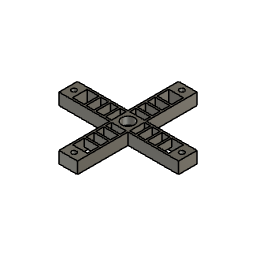
gripper v1 (Autodesk Fusion 360 design; units mm, degrees)
Autodesk Fusion 360 part; units mm, degrees
sketch "Esboço1" plane through (0, 0, 0) normal (0, 0, 1) x (1, 0, 0)
  line L0 (9.5, 9.5) -> (-9.5, 9.5)
  line L1 (-9.5, 9.5) -> (-9.5, -9.5)
  line L2 (-9.5, -9.5) -> (9.5, -9.5)
  line L3 (9.5, -9.5) -> (9.5, 9.5)
  line L4 (9.5, 9.5) -> (-9.5, -9.5) construction
  line L5 (-9.5, 9.5) -> (9.5, -9.5) construction
  circle A0 centre (0, 0) radius 6.5
  line L6 (-9.5, 9.5) -> (-7.5, 9.5)
  line L7 (-7.5, 9.5) -> (-7.5, 7.5)
  line L8 (-7.5, 7.5) -> (-9.5, 7.5)
  line L9 (-9.5, 7.5) -> (-9.5, 9.5)
  line L10 (9.5, 9.5) -> (7.5, 9.5)
  line L11 (7.5, 9.5) -> (7.5, 7.5)
  line L12 (7.5, 7.5) -> (9.5, 7.5)
  line L13 (9.5, 7.5) -> (9.5, 9.5)
  line L14 (-9.5, -9.5) -> (-7.5, -9.5)
  line L15 (-7.5, -9.5) -> (-7.5, -7.5)
  line L16 (-7.5, -7.5) -> (-9.5, -7.5)
  line L17 (-9.5, -7.5) -> (-9.5, -9.5)
  line L18 (9.5, -9.5) -> (7.5, -9.5)
  line L19 (7.5, -9.5) -> (7.5, -7.5)
  line L20 (7.5, -7.5) -> (9.5, -7.5)
  line L21 (9.5, -7.5) -> (9.5, -9.5)
  line L22 (-9.5, 9.5) -> (-7.5, 9.5)
  line L23 (-7.5, 9.5) -> (-7.5, 49.5)
  line L24 (-7.5, 49.5) -> (-9.5, 49.5)
  line L25 (-9.5, 49.5) -> (-9.5, 9.5)
  line L26 (9.5, 9.5) -> (7.5, 9.5)
  line L27 (7.5, 9.5) -> (7.5, 49.5)
  line L28 (7.5, 49.5) -> (9.5, 49.5)
  line L29 (9.5, 49.5) -> (9.5, 9.5)
  line L30 (-9.5, 49.5) -> (9.5, 49.5)
  line L31 (9.5, 49.5) -> (9.5, 61.5)
  line L32 (9.5, 61.5) -> (-9.5, 61.5)
  line L33 (-9.5, 61.5) -> (-9.5, 49.5)
  line L34 (-9.5, 61.5) -> (9.5, 49.5) construction
  circle A1 centre (0, 55.5) radius 2.5
  line L35 (-7.5, 9.5) -> (7.5, 9.5)
  line L36 (7.5, 9.5) -> (7.5, 15.5)
  line L37 (7.5, 15.5) -> (-7.5, 15.5)
  line L38 (-7.5, 15.5) -> (-7.5, 9.5)
  line L39 (-7.5, 15.5) -> (7.5, 15.5)
  line L40 (7.5, 15.5) -> (7.5, 17.5)
  line L41 (7.5, 17.5) -> (-7.5, 17.5)
  line L42 (-7.5, 17.5) -> (-7.5, 15.5)
  line L43 (-7.5, 17.5) -> (7.5, 17.5)
  line L44 (7.5, 17.5) -> (7.5, 25.5)
  line L45 (7.5, 25.5) -> (-7.5, 25.5)
  line L46 (-7.5, 25.5) -> (-7.5, 17.5)
  line L47 (-7.5, 25.5) -> (7.5, 25.5)
  line L48 (7.5, 25.5) -> (7.5, 27.5)
  line L49 (7.5, 27.5) -> (-7.5, 27.5)
  line L50 (-7.5, 27.5) -> (-7.5, 25.5)
  line L51 (-7.5, 27.5) -> (7.5, 27.5)
  line L52 (7.5, 27.5) -> (7.5, 35.5)
  line L53 (7.5, 35.5) -> (-7.5, 35.5)
  line L54 (-7.5, 35.5) -> (-7.5, 27.5)
  line L55 (-7.5, 35.5) -> (7.5, 35.5)
  line L56 (7.5, 35.5) -> (7.5, 37.5)
  line L57 (7.5, 37.5) -> (-7.5, 37.5)
  line L58 (-7.5, 37.5) -> (-7.5, 35.5)
  line L59 (9.5, 9.5) -> (49.5, 9.5)
  line L60 (49.5, 9.5) -> (49.5, 7.5)
  line L61 (49.5, 7.5) -> (9.5, 7.5)
  line L62 (9.5, 7.5) -> (9.5, 9.5)
  line L63 (9.5, -9.5) -> (49.5, -9.5)
  line L64 (49.5, -9.5) -> (49.5, -7.5)
  line L65 (49.5, -7.5) -> (9.5, -7.5)
  line L66 (9.5, -7.5) -> (9.5, -9.5)
  line L67 (49.5, 9.5) -> (61.5, 9.5)
  line L68 (61.5, 9.5) -> (61.5, -9.5)
  line L69 (61.5, -9.5) -> (49.5, -9.5)
  line L70 (49.5, -9.5) -> (49.5, 9.5)
  line L71 (49.5, 9.5) -> (61.5, -9.5) construction
  circle A2 centre (55.5, 0) radius 2.5
  line L72 (9.5, 7.5) -> (15.5, 7.5)
  line L73 (15.5, 7.5) -> (15.5, -7.5)
  line L74 (15.5, -7.5) -> (9.5, -7.5)
  line L75 (9.5, -7.5) -> (9.5, 7.5)
  line L76 (15.5, 7.5) -> (17.5, 7.5)
  line L77 (17.5, 7.5) -> (17.5, -7.5)
  line L78 (17.5, -7.5) -> (15.5, -7.5)
  line L79 (15.5, -7.5) -> (15.5, 7.5)
  line L80 (17.5, 7.5) -> (25.5, 7.5)
  line L81 (25.5, 7.5) -> (25.5, -7.5)
  line L82 (25.5, -7.5) -> (17.5, -7.5)
  line L83 (17.5, -7.5) -> (17.5, 7.5)
  line L84 (25.5, 7.5) -> (27.5, 7.5)
  line L85 (27.5, 7.5) -> (27.5, -7.5)
  line L86 (27.5, -7.5) -> (25.5, -7.5)
  line L87 (25.5, -7.5) -> (25.5, 7.5)
  line L88 (27.5, 7.5) -> (35.5, 7.5)
  line L89 (35.5, 7.5) -> (35.5, -7.5)
  line L90 (35.5, -7.5) -> (27.5, -7.5)
  line L91 (27.5, -7.5) -> (27.5, 7.5)
  line L92 (35.5, 7.5) -> (37.5, 7.5)
  line L93 (37.5, 7.5) -> (37.5, -7.5)
  line L94 (37.5, -7.5) -> (35.5, -7.5)
  line L95 (35.5, -7.5) -> (35.5, 7.5)
  line L96 (-9.5, -9.5) -> (-7.5, -9.5)
  line L97 (-7.5, -9.5) -> (-7.5, -49.5)
  line L98 (-7.5, -49.5) -> (-9.5, -49.5)
  line L99 (-9.5, -49.5) -> (-9.5, -9.5)
  line L100 (9.5, -9.5) -> (7.5, -9.5)
  line L101 (7.5, -9.5) -> (7.5, -49.5)
  line L102 (7.5, -49.5) -> (9.5, -49.5)
  line L103 (9.5, -49.5) -> (9.5, -9.5)
  line L104 (-9.5, -49.5) -> (9.5, -49.5)
  line L105 (9.5, -49.5) -> (9.5, -61.5)
  line L106 (9.5, -61.5) -> (-9.5, -61.5)
  line L107 (-9.5, -61.5) -> (-9.5, -49.5)
  line L108 (-9.5, -49.5) -> (9.5, -61.5) construction
  circle A3 centre (0, -55.5) radius 2.5
  line L109 (-9.5, -9.5) -> (9.5, -9.5)
  line L110 (9.5, -9.5) -> (9.5, -15.5)
  line L111 (9.5, -15.5) -> (-9.5, -15.5)
  line L112 (-9.5, -15.5) -> (-9.5, -9.5)
  line L113 (-9.5, -15.5) -> (9.5, -15.5)
  line L114 (9.5, -15.5) -> (9.5, -17.5)
  line L115 (9.5, -17.5) -> (-9.5, -17.5)
  line L116 (-9.5, -17.5) -> (-9.5, -15.5)
  line L117 (-9.5, -17.5) -> (9.5, -17.5)
  line L118 (9.5, -17.5) -> (9.5, -25.5)
  line L119 (9.5, -25.5) -> (-9.5, -25.5)
  line L120 (-9.5, -25.5) -> (-9.5, -17.5)
  line L121 (-9.5, -25.5) -> (9.5, -25.5)
  line L122 (9.5, -25.5) -> (9.5, -27.5)
  line L123 (9.5, -27.5) -> (-9.5, -27.5)
  line L124 (-9.5, -27.5) -> (-9.5, -25.5)
  line L125 (-9.5, -27.5) -> (9.5, -27.5)
  line L126 (9.5, -27.5) -> (9.5, -35.5)
  line L127 (9.5, -35.5) -> (-9.5, -35.5)
  line L128 (-9.5, -35.5) -> (-9.5, -27.5)
  line L129 (-9.5, -35.5) -> (9.5, -35.5)
  line L130 (9.5, -35.5) -> (9.5, -37.5)
  line L131 (9.5, -37.5) -> (-9.5, -37.5)
  line L132 (-9.5, -37.5) -> (-9.5, -35.5)
  line L133 (-9.5, 9.5) -> (-49.5, 9.5)
  line L134 (-49.5, 9.5) -> (-49.5, 7.5)
  line L135 (-49.5, 7.5) -> (-9.5, 7.5)
  line L136 (-9.5, 7.5) -> (-9.5, 9.5)
  line L137 (-9.5, -9.5) -> (-49.5, -9.5)
  line L138 (-49.5, -9.5) -> (-49.5, -7.5)
  line L139 (-49.5, -7.5) -> (-9.5, -7.5)
  line L140 (-9.5, -7.5) -> (-9.5, -9.5)
  line L141 (-49.5, -9.5) -> (-61.5, -9.5)
  line L142 (-61.5, -9.5) -> (-61.5, 9.5)
  line L143 (-61.5, 9.5) -> (-49.5, 9.5)
  line L144 (-49.5, 9.5) -> (-49.5, -9.5)
  line L145 (-61.5, 9.5) -> (-49.5, -9.5) construction
  circle A4 centre (-55.5, 0) radius 2.5
  line L146 (-9.5, 9.5) -> (-15.5, 9.5)
  line L147 (-15.5, 9.5) -> (-15.5, -9.5)
  line L148 (-15.5, -9.5) -> (-9.5, -9.5)
  line L149 (-9.5, -9.5) -> (-9.5, 9.5)
  line L150 (-15.5, 9.5) -> (-17.5, 9.5)
  line L151 (-17.5, 9.5) -> (-17.5, -9.5)
  line L152 (-17.5, -9.5) -> (-15.5, -9.5)
  line L153 (-15.5, -9.5) -> (-15.5, 9.5)
  line L154 (-17.5, 9.5) -> (-25.5, 9.5)
  line L155 (-25.5, 9.5) -> (-25.5, -9.5)
  line L156 (-25.5, -9.5) -> (-17.5, -9.5)
  line L157 (-17.5, -9.5) -> (-17.5, 9.5)
  line L158 (-25.5, 9.5) -> (-27.5, 9.5)
  line L159 (-27.5, 9.5) -> (-27.5, -9.5)
  line L160 (-27.5, -9.5) -> (-25.5, -9.5)
  line L161 (-25.5, -9.5) -> (-25.5, 9.5)
  line L162 (-27.5, 9.5) -> (-35.5, 9.5)
  line L163 (-35.5, 9.5) -> (-35.5, -9.5)
  line L164 (-35.5, -9.5) -> (-27.5, -9.5)
  line L165 (-27.5, -9.5) -> (-27.5, 9.5)
  line L166 (-35.5, 9.5) -> (-37.5, 9.5)
  line L167 (-37.5, 9.5) -> (-37.5, -9.5)
  line L168 (-37.5, -9.5) -> (-35.5, -9.5)
  line L169 (-35.5, -9.5) -> (-35.5, 9.5)
  dimension "d1" = 19
  dimension "d2" = 19
  dimension "d3" = 13
  dimension "d4" = 2
  dimension "d5" = 2
  dimension "d6" = 2
  dimension "d7" = 2
  dimension "d8" = 2
  dimension "d9" = 2
  dimension "d10" = 2
  dimension "d11" = 2
  dimension "d13" = 2
  dimension "d14" = 40
  dimension "d15" = 2
  dimension "d16" = 40
  dimension "d17" = 19
  dimension "d18" = 12
  dimension "d19" = 5
  dimension "d20" = 15
  dimension "d21" = 6
  dimension "d22" = 2
  dimension "d23" = 8
  dimension "d24" = 2
  dimension "d25" = 8
  dimension "d26" = 2
  dimension "d27" = 40
  dimension "d28" = 2
  dimension "d29" = 40
  dimension "d30" = 2
  dimension "d31" = 12
  dimension "d32" = 19
  dimension "d33" = 5
  dimension "d34" = 6
  dimension "d35" = 2
  dimension "d36" = 8
  dimension "d37" = 15
  dimension "d38" = 2
  dimension "d39" = 8
  dimension "d40" = 2
  dimension "d41" = 40
  dimension "d42" = 2
  dimension "d43" = 40
  dimension "d44" = 12
  dimension "d45" = 5
  dimension "d46" = 6
  dimension "d47" = 2
  dimension "d48" = 8
  dimension "d49" = 2
  dimension "d50" = 8
  dimension "d51" = 2
  dimension "d52" = 40
  dimension "d53" = 2
  dimension "d54" = 40
  dimension "d55" = 2
  dimension "d56" = 12
  dimension "d57" = 19
  dimension "d58" = 5
  dimension "d59" = 6
  dimension "d60" = 2
  dimension "d61" = 8
  dimension "d62" = 2
  dimension "d63" = 8
  dimension "d64" = 2
  constraint horizontal L0
  constraint perpendicular L0 L1
  constraint parallel L0 L2
  constraint parallel L1 L3
  constraint coincident L4 A0.centre
  constraint coincident L5 A0.centre
  constraint coincident A0.centre origin
  constraint horizontal L6
  constraint vertical L7
  constraint horizontal L8
  constraint vertical L9
  constraint horizontal L10
  constraint vertical L11
  constraint horizontal L12
  constraint vertical L13
  constraint horizontal L14
  constraint vertical L15
  constraint horizontal L16
  constraint vertical L17
  constraint horizontal L18
  constraint vertical L19
  constraint horizontal L20
  constraint vertical L21
  constraint horizontal L22
  constraint vertical L23
  constraint horizontal L24
  constraint vertical L25
  constraint horizontal L26
  constraint vertical L27
  constraint horizontal L28
  constraint vertical L29
  constraint horizontal L30
  constraint vertical L31
  constraint horizontal L32
  constraint vertical L33
  constraint midpoint L34 A1.centre
  constraint horizontal L35
  constraint vertical L36
  constraint horizontal L37
  constraint vertical L38
  constraint horizontal L39
  constraint vertical L40
  constraint horizontal L41
  constraint vertical L42
  constraint horizontal L43
  constraint vertical L44
  constraint horizontal L45
  constraint vertical L46
  constraint horizontal L47
  constraint vertical L48
  constraint horizontal L49
  constraint vertical L50
  constraint horizontal L51
  constraint vertical L52
  constraint horizontal L53
  constraint vertical L54
  constraint horizontal L55
  constraint vertical L56
  constraint horizontal L57
  constraint vertical L58
  constraint coincident L27 L56.end
  constraint horizontal L59
  constraint vertical L60
  constraint horizontal L61
  constraint vertical L62
  constraint horizontal L63
  constraint vertical L64
  constraint horizontal L65
  constraint vertical L66
  constraint horizontal L67
  constraint vertical L68
  constraint horizontal L69
  constraint vertical L70
  constraint midpoint L71 A2.centre
  constraint horizontal L72
  constraint vertical L73
  constraint horizontal L74
  constraint vertical L75
  constraint horizontal L76
  constraint vertical L77
  constraint horizontal L78
  constraint vertical L79
  constraint horizontal L80
  constraint vertical L81
  constraint horizontal L82
  constraint vertical L83
  constraint horizontal L84
  constraint vertical L85
  constraint horizontal L86
  constraint vertical L87
  constraint horizontal L88
  constraint vertical L89
  constraint horizontal L90
  constraint vertical L91
  constraint horizontal L92
  constraint vertical L93
  constraint horizontal L94
  constraint vertical L95
  constraint horizontal L96
  constraint vertical L97
  constraint horizontal L98
  constraint vertical L99
  constraint horizontal L100
  constraint vertical L101
  constraint horizontal L102
  constraint vertical L103
  constraint horizontal L104
  constraint vertical L105
  constraint horizontal L106
  constraint vertical L107
  constraint midpoint L108 A3.centre
  constraint horizontal L109
  constraint vertical L110
  constraint horizontal L111
  constraint vertical L112
  constraint horizontal L113
  constraint vertical L114
  constraint horizontal L115
  constraint vertical L116
  constraint horizontal L117
  constraint vertical L118
  constraint horizontal L119
  constraint vertical L120
  constraint horizontal L121
  constraint vertical L122
  constraint horizontal L123
  constraint vertical L124
  constraint horizontal L125
  constraint vertical L126
  constraint horizontal L127
  constraint vertical L128
  constraint horizontal L129
  constraint vertical L130
  constraint horizontal L131
  constraint vertical L132
  constraint horizontal L133
  constraint vertical L134
  constraint horizontal L135
  constraint vertical L136
  constraint horizontal L137
  constraint vertical L138
  constraint horizontal L139
  constraint vertical L140
  constraint horizontal L141
  constraint vertical L142
  constraint horizontal L143
  constraint vertical L144
  constraint midpoint L145 A4.centre
  constraint horizontal L146
  constraint vertical L147
  constraint horizontal L148
  constraint vertical L149
  constraint horizontal L150
  constraint vertical L151
  constraint horizontal L152
  constraint vertical L153
  constraint horizontal L154
  constraint vertical L155
  constraint horizontal L156
  constraint vertical L157
  constraint horizontal L158
  constraint vertical L159
  constraint horizontal L160
  constraint vertical L161
  constraint horizontal L162
  constraint vertical L163
  constraint horizontal L164
  constraint vertical L165
  constraint horizontal L166
  constraint vertical L167
  constraint horizontal L168
  constraint vertical L169
  measures "d1" distance of L1.end L2.end
  measures "d2" distance of L0.start L2.end
  measures "d3" diameter of A0
  measures "d4" distance of L0.end L6.end
  measures "d5" distance of L0.end L8.end
  measures "d6" distance of L0.start L10.end
  measures "d7" distance of L0.start L12.end
  measures "d8" distance of L1.end L14.end
  measures "d9" distance of L1.end L16.end
  measures "d10" distance of L2.end L18.end
  measures "d11" distance of L2.end L20.end
  measures "d13" distance of L0.end L6.end
  measures "d14" distance of L0.end L24.end
  measures "d15" distance of L0.start L10.end
  measures "d16" distance of L0.start L28.end
  measures "d17" distance of L24.end L28.end
  measures "d18" distance of L24.end L32.end
  measures "d19" diameter of A1
  measures "d20" distance of L6.end L10.end
  measures "d21" distance of L6.end L37.end
  measures "d22" distance of L37.end L41.end
  measures "d23" distance of L41.end L45.end
  measures "d24" distance of L45.end L49.end
  measures "d25" distance of L49.end L53.end
  measures "d26" distance of L53.end L57.end
  measures "d27" distance of L0.start L59.end
  measures "d28" distance of L0.start L12.end
  measures "d29" distance of L2.end L63.end
  measures "d30" distance of L2.end L20.end
  measures "d31" distance of L59.end L67.end
  measures "d32" distance of L59.end L63.end
  measures "d33" diameter of A2
  measures "d34" distance of L12.end L72.end
  measures "d35" distance of L72.end L76.end
  measures "d36" distance of L76.end L80.end L9
  measures "d37" distance of L76.end L77.end L9
  measures "d38" distance of L80.end L84.end
  measures "d39" distance of L84.end L88.end L9
  measures "d40" distance of L88.end L92.end
  measures "d41" distance of L1.end L98.end
  measures "d42" distance of L2.end L18.end
  measures "d43" distance of L2.end L102.end
  measures "d44" distance of L98.end L106.end
  measures "d45" diameter of A3
  measures "d46" distance of L1.end L111.end
  measures "d47" distance of L111.end L115.end
  measures "d48" distance of L115.end L119.end
  measures "d49" distance of L119.end L123.end
  measures "d50" distance of L123.end L127.end
  measures "d51" distance of L127.end L131.end
  measures "d52" distance of L0.end L133.end
  measures "d53" distance of L0.end L8.end
  measures "d54" distance of L1.end L137.end
  measures "d55" distance of L1.end L16.end
  measures "d56" distance of L137.end L141.end
  measures "d57" distance of L137.end L133.end
  measures "d58" diameter of A4
  measures "d59" distance of L0.end L146.end
  measures "d60" distance of L146.end L150.end
  measures "d61" distance of L150.end L154.end
  measures "d62" distance of L154.end L158.end
  measures "d63" distance of L158.end L162.end
  measures "d64" distance of L162.end L166.end
extrude "Extrusão1" add sketch "Esboço1" along normal blind 8 contours L0 L3 L10 L11 L12 L13 L26 L62 | L3 L13 L59 L60 L61 L62 L70 L72 L76 L80 L84 L88 L92 | L0 L10 L26 L27 L28 L29 L30 L36 L40 L44 L48 L52 L56 | L0 L1 L2 L3 L7 L8 L11 L12 L15 L16 L19 L20 L35 L75 L109 L149 | L24 L28 L30 L31 L32 L33 | L60 L64 L67 L68 L69 L70 | L0 L1 L6 L7 L8 L9 L22 L136 L149 | L0 L6 L22 L23 L24 L25 L30 L38 L42 L46 L50 L54 L58 | L23 L27 L37 L39 L40 L41 L42 L43 | L3 L21 L63 L64 L65 L66 L70 L74 L78 L82 L86 L90 L94 | L2 L3 L18 L19 L20 L21 L66 L100 L109 | L61 L65 L73 L76 L77 L78 L79 L83 | L1 L9 L133 L135 L136 L146 L147 L149 L153 | L2 L18 L100 L101 L103 L109 L110 L111 L113 | L23 L27 L53 L55 L56 L57 L58 | L61 L65 L89 L92 L93 L94 L95 | L133 L135 L147 L150 L151 L153 L157 | L23 L27 L45 L47 L48 L49 L50 L51 | L101 L103 L111 L113 L114 L115 L117 | L61 L65 L81 L84 L85 L86 L87 L91 | L1 L2 L14 L15 L16 L17 L96 L109 L140 L149 | L1 L17 L137 L139 L140 L147 L148 L149 L153 | L135 L139 L147 L151 L153 L157 | L133 L135 L151 L154 L155 L157 L161 | L2 L14 L96 L97 L99 L109 L111 L112 L113 | L97 L101 L111 L113 L115 L117 | L101 L103 L115 L117 L118 L119 L121 | L137 L139 L147 L151 L152 L153 L157 | L133 L135 L155 L158 L159 L161 L165 | L97 L99 L111 L113 L115 L116 L117 | L101 L103 L119 L121 L122 L123 L125 | L137 L139 L151 L155 L156 L157 L161 | L135 L139 L155 L159 L161 L165 | L133 L135 L159 L162 L163 L165 L169 | L97 L99 L115 L117 L119 L120 L121 | L97 L101 L119 L121 L123 L125 | L101 L103 L123 L125 L126 L127 L129 | L137 L139 L155 L159 L160 L161 L165 | L133 L135 L163 L166 L167 L169 | L97 L99 L119 L121 L123 L124 L125 | L101 L103 L127 L129 L130 L131 | L137 L139 L159 L163 L164 L165 L169 | L135 L139 L163 L167 L169 | L133 L134 L135 L144 L167 | L97 L99 L123 L125 L127 L128 L129 | L97 L101 L127 L129 L131 | L101 L102 L103 L104 L131 | L137 L139 L163 L167 L168 L169 | L134 L138 L141 L142 L143 L144 | L97 L99 L127 L129 L131 L132 | L98 L102 L104 L105 L106 L107 | L137 L138 L139 L144 L167 | L97 L98 L99 L104 L131
extrude "Extrusão2" add sketch "Esboço1" against normal blind 4 contours L0 L3 L10 L11 L12 L13 L26 L62 | L3 L13 L59 L60 L61 L62 L70 L72 L76 L80 L84 L88 L92 | L0 L10 L26 L27 L28 L29 L30 L36 L40 L44 L48 L52 L56 | L24 L28 L30 L31 L32 L33 | L60 L64 L67 L68 L69 L70 | L0 L1 L6 L7 L8 L9 L22 L136 L149 | L0 L6 L22 L23 L24 L25 L30 L38 L42 L46 L50 L54 L58 | L3 L21 L63 L64 L65 L66 L70 L74 L78 L82 L86 L90 L94 | L2 L3 L18 L19 L20 L21 L66 L100 L109 | L1 L9 L133 L135 L136 L146 L147 L149 L153 | L2 L18 L100 L101 L103 L109 L110 L111 L113 | L133 L135 L147 L150 L151 L153 L157 | L101 L103 L111 L113 L114 L115 L117 | L1 L2 L14 L15 L16 L17 L96 L109 L140 L149 | L1 L17 L137 L139 L140 L147 L148 L149 L153 | L133 L135 L151 L154 L155 L157 L161 | L2 L14 L96 L97 L99 L109 L111 L112 L113 | L101 L103 L115 L117 L118 L119 L121 | L137 L139 L147 L151 L152 L153 L157 | L133 L135 L155 L158 L159 L161 L165 | L97 L99 L111 L113 L115 L116 L117 | L101 L103 L119 L121 L122 L123 L125 | L137 L139 L151 L155 L156 L157 L161 | L133 L135 L159 L162 L163 L165 L169 | L97 L99 L115 L117 L119 L120 L121 | L101 L103 L123 L125 L126 L127 L129 | L137 L139 L155 L159 L160 L161 L165 | L133 L135 L163 L166 L167 L169 | L97 L99 L119 L121 L123 L124 L125 | L101 L103 L127 L129 L130 L131 | L137 L139 L159 L163 L164 L165 L169 | L133 L134 L135 L144 L167 | L97 L99 L123 L125 L127 L128 L129 | L101 L102 L103 L104 L131 | L137 L139 L163 L167 L168 L169 | L134 L138 L141 L142 L143 L144 | L97 L99 L127 L129 L131 L132 | L98 L102 L104 L105 L106 L107 | L137 L138 L139 L144 L167 | L97 L98 L99 L104 L131
